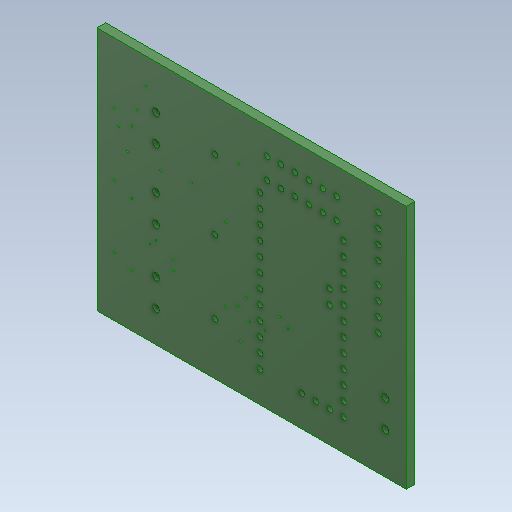
# Autodesk Inventor part: dog_driver_5.brd_Outline
Saved by Autodesk Inventor 2020 (Build 240168000, 168)
## iProperties
Created: 2019-08-29
Part Number: dog_driver_5.brd_Outline
Material: Generic
Document SubType Name: Modeling
Designer: psrob
Density: 1 g/cm^3
Appearance: Board Outline
Author: psrob
Autodesk Inventor part; units mm, degrees
ref_plane "YZ Plane" through (0, 0, 0) normal (1, 0, 0) x (0, 1, 0)
ref_plane "XZ Plane" through (0, 0, 0) normal (0, 1, 0) x (-1, 0, 0)
ref_plane "XY Plane" through (0, 0, 0) normal (0, 0, 1) x (1, 0, 0)
sketch "Sketch1" plane through (0, 0, 0) normal (0, 0, 1) x (1, 0, 0)
  line L0 (0.635, 3.175) -> (57.13, 3.175)
  line L1 (57.13, 3.175) -> (57.13, 47.93)
  line L2 (57.13, 47.93) -> (0.635, 47.93)
  line L3 (0.635, 47.93) -> (0.635, 3.175)
  circle A0 centre (45.72, 19.05) radius 0.5
  circle A1 centre (45.72, 21.59) radius 0.5
  circle A2 centre (45.72, 24.13) radius 0.5
  circle A3 centre (45.72, 26.67) radius 0.5
  circle A4 centre (43.18, 25.4) radius 0.5
  circle A5 centre (43.18, 27.94) radius 0.5
  circle A6 centre (40.64, 8.89) radius 0.5
  circle A7 centre (43.18, 8.89) radius 0.5
  circle A8 centre (44.45, 39.37) radius 0.5
  circle A9 centre (30.48, 26.67) radius 0.5
  circle A10 centre (30.48, 24.13) radius 0.5
  circle A11 centre (30.48, 21.59) radius 0.5
  circle A12 centre (30.48, 19.05) radius 0.5
  circle A13 centre (30.48, 16.51) radius 0.5
  circle A14 centre (30.48, 13.97) radius 0.5
  circle A15 centre (30.48, 11.43) radius 0.5
  circle A16 centre (30.48, 8.89) radius 0.5
  circle A17 centre (45.72, 8.89) radius 0.5
  circle A18 centre (45.72, 11.43) radius 0.5
  circle A19 centre (45.72, 13.97) radius 0.5
  circle A20 centre (45.72, 16.51) radius 0.5
  circle A21 centre (31.75, 39.37) radius 0.5
  circle A22 centre (30.48, 29.21) radius 0.5
  circle A23 centre (45.72, 34.29) radius 0.5
  circle A24 centre (41.91, 39.37) radius 0.5
  circle A25 centre (38.1, 8.89) radius 0.5
  circle A26 centre (45.72, 36.83) radius 0.5
  circle A27 centre (45.72, 31.75) radius 0.5
  circle A28 centre (30.48, 31.75) radius 0.5
  circle A29 centre (30.48, 34.29) radius 0.5
  circle A30 centre (36.83, 39.37) radius 0.5
  circle A31 centre (30.48, 36.83) radius 0.5
  circle A32 centre (34.29, 39.37) radius 0.5
  circle A33 centre (45.72, 29.21) radius 0.5
  circle A34 centre (39.37, 39.37) radius 0.5
  circle A35 centre (11.43, 13.97) radius 0.65
  circle A36 centre (11.43, 8.97) radius 0.65
  circle A37 centre (11.43, 27.3) radius 0.65
  circle A38 centre (11.43, 22.3) radius 0.65
  circle A39 centre (11.43, 40.01) radius 0.65
  circle A40 centre (11.43, 35.01) radius 0.65
  circle A41 centre (53.34, 10.79) radius 0.65
  circle A42 centre (53.34, 15.79) radius 0.65
  circle A43 centre (44.45, 43.18) radius 0.51
  circle A44 centre (41.91, 43.18) radius 0.51
  circle A45 centre (39.37, 43.18) radius 0.51
  circle A46 centre (36.83, 43.18) radius 0.51
  circle A47 centre (34.29, 43.18) radius 0.51
  circle A48 centre (31.75, 43.18) radius 0.51
  circle A49 centre (52.07, 44.45) radius 0.51
  circle A50 centre (52.07, 41.91) radius 0.51
  circle A51 centre (52.07, 39.37) radius 0.51
  circle A52 centre (52.07, 36.83) radius 0.51
  circle A53 centre (52.07, 33.02) radius 0.51
  circle A54 centre (52.07, 30.48) radius 0.51
  circle A55 centre (52.07, 27.94) radius 0.51
  circle A56 centre (52.07, 25.4) radius 0.51
  circle A57 centre (3.81, 36.83) radius 0.175
  circle A58 centre (3.81, 25.4) radius 0.175
  circle A59 centre (3.81, 13.97) radius 0.175
  circle A60 centre (9.525, 43.18) radius 0.175
  circle A61 centre (24.13, 15.5575) radius 0.175
  circle A62 centre (24.13, 28.8925) radius 0.175
  circle A63 centre (22.225, 38.735) radius 0.5
  circle A64 centre (22.225, 26.035) radius 0.5
  circle A65 centre (22.225, 12.7) radius 0.5
  circle A66 centre (6.985, 35.56) radius 0.175
  circle A67 centre (6.985, 24.13) radius 0.175
  circle A68 centre (6.985, 12.7) radius 0.175
  circle A69 centre (8.001, 38.608) radius 0.175
  circle A70 centre (17.9388, 32.0675) radius 0.175
  circle A71 centre (12.2238, 31.115) radius 0.175
  circle A72 centre (28.575, 15.3988) radius 0.175
  circle A73 centre (31.2738, 15.3988) radius 0.175
  circle A74 centre (27.94, 18.8912) radius 0.175
  circle A75 centre (26.3525, 16.8275) radius 0.175
  circle A76 centre (26.5113, 39.37) radius 0.175
  circle A77 centre (14.605, 16.51) radius 0.175
  circle A78 centre (14.605, 18.1588) radius 0.175
  circle A79 centre (10.3096, 18.6032) radius 0.175
  circle A80 centre (11.43, 19.685) radius 0.175
  circle A81 centre (26.8288, 11.43) radius 0.175
  circle A82 centre (33.9725, 18.8912) radius 0.175
  circle A83 centre (4.5946, 34.29) radius 0.175
  circle A84 centre (6.2004, 31.115) radius 0.175
  circle A85 centre (35.56, 17.78) radius 0.175
  constraints: 86 centre point, 8 end point
extrude "dog_driver_5.brd_Outline" add sketch "Sketch1" along normal blind 1.6
body "Solid1"
